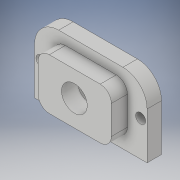
# Autodesk Inventor part: Aquamote3.2_housing_cap
Saved by Autodesk Inventor 2018 (Build 220112000, 112)
## iProperties
Created: 2018-04-23
Part Number: Aquamote3.2_housing_cap
Material: Generic
Document SubType Name: Modeling
Designer: Leon
Density: 1 g/cm^3
Appearance: Default
Author: Leon
Autodesk Inventor part; units mm, degrees
ref_plane "YZ Plane" through (0, 0, 0) normal (1, 0, 0) x (0, 1, 0)
ref_plane "XZ Plane" through (0, 0, 0) normal (0, 1, 0) x (-1, 0, 0)
ref_plane "XY Plane" through (0, 0, 0) normal (0, 0, 1) x (1, 0, 0)
sketch "Sketch1" plane through (0, 0, 0) normal (0, 0, 1) x (1, 0, 0)
  line L0 (0, 0) -> (35, 0)
  line L1 (35, 0) -> (35, 14.5)
  line L2 (27.5, 22) -> (7.5, 22)
  line L3 (0, 14.5) -> (0, 0)
  arc A0 (7.5, 22) -> (0, 14.5) centre (7.5, 14.5) ccw
  arc A1 (35, 14.5) -> (27.5, 22) centre (27.5, 14.5) ccw
  point P0 (35, 22)
  point P1 (0, 22)
  dimension "d0" = 35
  dimension "d1" = 22
  dimension "d2" = 7.5
  constraints: 8 end point, 4 point on circle, 4 point on line, 4 tangent, 2 centre point, 2 parallel, 1 equal radius, 1 horizontal, 1 perpendicular
  measures "d0" distance of point (0, 22) point (35, 22)
  measures "d1" distance of point (35, 22) L0.end
  measures "d2" radius of A0
extrude "Extrusion1" add sketch "Sketch1" along normal blind 4.5
sketch "Sketch2" plane through (0, 0, 4.5) normal (0, 0, 1) x (1, 0, 0)
  line L0 (9.5807, 3.0793) -> (25.4203, 3.0793)
  line L1 (28.8863, 6.5453) -> (28.8863, 15.4547)
  line L2 (25.4203, 18.9207) -> (9.5807, 18.9207)
  line L3 (6.1147, 15.4547) -> (6.1147, 6.5453)
  arc A0 (9.5807, 18.9207) -> (6.1147, 15.4547) centre (9.5807, 15.4547) ccw
  arc A1 (28.8863, 15.4547) -> (25.4203, 18.9207) centre (25.4203, 15.4547) ccw
  arc A2 (25.4203, 3.0793) -> (28.8863, 6.5453) centre (25.4203, 6.5453) ccw
  arc A3 (6.1147, 6.5453) -> (9.5807, 3.0793) centre (9.5807, 6.5453) ccw
  line L4 (35, 0) -> (35, 14.5) projected
  line L5 (0, 0) -> (35, 0) projected
  line L6 (0, 14.5) -> (0, 0) projected
  line L7 (27.5, 22) -> (7.5, 22) projected
  point P0 (29, 19)
  point P1 (29, 3)
  point P2 (6, 19)
  dimension "d5" = 23
  dimension "d6" = 16
  dimension "d7" = 3.466
  dimension "d8" = 3.466
  dimension "d9" = 6.1137
  dimension "d10" = 3.0793
  dimension "d49" = 6.1147
  dimension "d50" = 3.0793
  constraints: 8 end point, 8 point on circle, 8 tangent, 4 centre point, 2 equal radius, 2 parallel, 1 horizontal, 1 perpendicular
  measures "d5" distance of point (6, 19) point (29, 19)
  measures "d6" distance of point (29, 19) point (29, 3)
  measures "d7" radius of A0
  measures "d8" radius of A3
  measures "d9" distance between parallel lines of L4 L1
  measures "d10" distance between parallel lines of L5 L0
  measures "d49" distance between parallel lines of L6 L3
  measures "d50" distance between parallel lines of L2 L7
extrude "Extrusion2" add sketch "Sketch2" along normal blind 5
sketch "Sketch3" plane through (0, 0, 0) normal (0, 0, -1) x (-1, 0, 0)
  circle A0 centre (-2, 11) radius 1.56
  circle A1 centre (-33, 11) radius 1.56
  line L0 (0, 14.5) -> (0, 0) projected
  line L1 (0, 0) -> (-35, 0) projected
  dimension "d13" = 3.12
  dimension "d14" = 3.12
  dimension "d18" = 2
  dimension "d19" = 31
  dimension "d20" = 11
  dimension "d21" = 11
  constraints: 2 centre point
  measures "d13" diameter of A0
  measures "d14" diameter of A1
  measures "d18" distance from line of L0 A0.centre
  measures "d19" distance of A1.centre A0.centre
  measures "d20" distance from line of L1 A1.centre
  measures "d21" distance from line of L1 A0.centre
hole "Hole1" at (2, 11, 0) direction (0, 0, 1) diameter 3.12 end through all
hole "Hole2" at (33, 11, 0) direction (0, 0, 1) diameter 3.12 end through all
sketch "Sketch4" plane through (0, 0, 9.5) normal (0, 0, 1) x (1, 0, 0)
  circle A0 centre (17.3863, 11.0793) radius 4
  line L0 (28.8863, 6.5453) -> (28.8863, 15.4547) projected
  line L1 (9.5807, 3.0793) -> (25.4203, 3.0793) projected
  point P0 (0, 0)
  dimension "d36" = 8
  dimension "d37" = 11.5
  dimension "d38" = 8
  constraints: 1 centre point
  measures "d36" diameter of A0
  measures "d37" distance from line of L0 A0.centre
  measures "d38" distance from line of L1 A0.centre
extrude "Extrusion3" cut sketch "Sketch4" against normal blind 5
sketch "Sketch5" plane through (17.3863, 11.0793, 4.5) normal (0, 0, 1) x (1, 0, 0)
  circle A0 centre (0, 0) radius 1.55
  circle A1 centre (0, 0) radius 4 projected
  point P0 (-17.3863, -11.0793)
  dimension "d41" = 3.1
  dimension "d42" = 2.45
  constraints: 1 centre point
  measures "d41" diameter of A0
  measures "d42" radial gap between concentric circles of A1 A0
extrude "Extrusion4" cut sketch "Sketch5" against normal blind 2.15 contours A0
sketch "Sketch6" plane through (17.3863, 11.0793, 2.35) normal (0, 0, 1) x (1, 0, 0)
  circle A0 centre (0.0058, 0.0144) radius 1.005
  circle A1 centre (0, 0) radius 1.55 projected
  point P0 (-17.3863, -11.0793)
  dimension "d45" = 2.01
  dimension "d46" = 0.5295
  constraints: 1 centre point
  measures "d45" diameter of A0
extrude "Extrusion5" cut sketch "Sketch6" against normal through all contours A0
body "Solid1"
